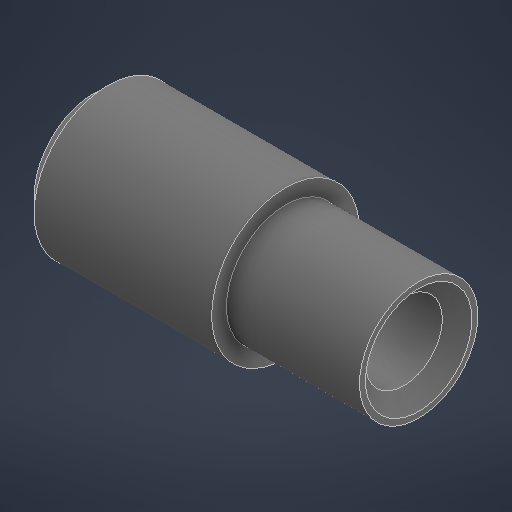
# Autodesk Inventor part: Vezetőhüvely
Saved by Autodesk Inventor 2025 (Build 290162010, 162A)
## iProperties
Created: 2025-02-13
Part Number: Vezetőhüvely
Material: Generic
Document SubType Name: Modeling
Designer: petruska.milan
Density: 1 g/cm^3
Appearance: Gray
Author: petruska.milan
Autodesk Inventor part; units mm, degrees
ref_plane "YZ Plane" through (0, 0, 0) normal (1, 0, 0) x (0, 1, 0)
ref_plane "XZ Plane" through (0, 0, 0) normal (0, 1, 0) x (-1, 0, 0)
ref_plane "XY Plane" through (0, 0, 0) normal (0, 0, 1) x (1, 0, 0)
sketch "Sketch1" plane through (0, 0, 0) normal (0, 0, 1) x (1, 0, 0)
  line L0 (0, 0) -> (22, 0)
  line L1 (22, 0) -> (22, 5)
  line L2 (22, 5) -> (0, 5)
  line L3 (0, 5) -> (0, 0)
  line L4 (22, 0) -> (13, 0)
  line L5 (13, 0) -> (13, 4)
  line L6 (13, 4) -> (22, 4)
  line L7 (22, 4) -> (22, 0)
  line L8 (13, 4) -> (13, 5)
  line L9 (22, 0) -> (0, 0)
  line L10 (0, 0) -> (0, 2.6)
  line L11 (0, 2.6) -> (22, 2.6)
  line L12 (22, 2.6) -> (22, 0)
  dimension "d0" = 22
  dimension "d1" = 5
  dimension "d2" = 9
  dimension "d3" = 4
  dimension "d4" = 2.6
  constraints: 26 end point, 6 parallel, 4 perpendicular, 3 horizontal, 2 point on line
  measures "d0" distance of L2.end L1.end
  measures "d1" distance of L2.end L0.start
  measures "d2" distance of L5.end L6.end
  measures "d3" distance of L4.end L5.end
  measures "d4" distance of L9.end L10.end
revolve "Revolution1" add sketch "Sketch1" angle 360 about axis through (0, 0, 0) along (1, 0, 0) contours L3 L2 L8 L5 L11 | L5 L6 L1 L11
chamfer "Chamfer1" distance 1 angle 45 3 edges at (22, -2.6, 0) (0, -2.6, 0) (0, -5, 0)
body "Solid1"
